Autodesk Inventor part; units mm, degrees
(part 2 of 2)
sketch "Sketch26" plane through (0, 0, 0) normal (0, -1, 0) x (1, 0, 0)
  circle A0 centre (0, 0) radius 23.8125 construction
  spline S0 degree 2 poles (-25.008, 3.6624) (-24.6681, 3.636) (-24.1674, 3.3369) (-24.0142, 3.1094) knots 0 0 0 1 2 2 2
  spline S1 degree 2 poles (-24.0142, 3.1094) (-23.8348, 2.8353) (-23.7106, 2.2348) (-23.7468, 1.7694) knots 0 0 0 1 2 2 2
  line L0 (-23.7468, 1.7694) -> (-23.8485, 0.4617)
  line L1 (-23.8485, 0.4617) -> (-28.4068, 0.8163)
  line L2 (-28.4068, 0.8163) -> (-28.3128, 2.0242)
  spline S2 degree 2 poles (-28.3128, 2.0242) (-28.2749, 2.5118) (-28.1741, 2.9945) (-28.035, 3.2067) knots 0 0 0 1 2 2 2
  spline S3 degree 2 poles (-28.035, 3.2067) (-27.8864, 3.4441) (-27.4441, 3.6364) (-27.156, 3.614) knots 0 0 0 1 2 2 2
  spline S4 degree 2 poles (-27.156, 3.614) (-26.8346, 3.589) (-26.3513, 3.2095) (-26.2305, 2.8991) knots 0 0 0 1 2 2 2
  line L3 (-26.2305, 2.8991) -> (-26.2084, 2.8973)
  spline S5 degree 2 poles (-26.2084, 2.8973) (-26.0659, 3.2951) (-25.4439, 3.6963) (-25.008, 3.6624) knots 0 0 0 1 2 2 2
  spline S6 degree 2 poles (-25.0313, 3.0287) (-25.2898, 3.0489) (-25.6338, 2.927) (-25.7692, 2.7145) knots 0 0 0 1 2 2 2
  spline S7 degree 2 poles (-25.7692, 2.7145) (-25.8543, 2.5762) (-25.9251, 2.2398) (-25.9495, 1.9259) knots 0 0 0 1 2 2 2
  line L4 (-25.9495, 1.9259) -> (-26.0029, 1.2388)
  line L5 (-26.0029, 1.2388) -> (-24.3185, 1.1078)
  line L6 (-24.3185, 1.1078) -> (-24.2803, 1.599)
  spline S8 degree 2 poles (-24.2803, 1.599) (-24.2493, 1.998) (-24.2875, 2.4618) (-24.3919, 2.6483) knots 0 0 0 1 2 2 2
  spline S9 degree 2 poles (-24.3919, 2.6483) (-24.5006, 2.8277) (-24.7912, 3.0101) (-25.0313, 3.0287) knots 0 0 0 1 2 2 2
  spline S10 degree 2 poles (-27.1202, 2.9757) (-27.2827, 2.9884) (-27.5351, 2.8965) (-27.6148, 2.7801) knots 0 0 0 1 2 2 2
  spline S11 degree 2 poles (-27.6148, 2.7801) (-27.7076, 2.6386) (-27.7724, 2.2832) (-27.7974, 1.9618) knots 0 0 0 1 2 2 2
  line L7 (-27.7974, 1.9618) -> (-27.8425, 1.3819)
  line L8 (-27.8425, 1.3819) -> (-26.509, 1.2782)
  line L9 (-26.509, 1.2782) -> (-26.4556, 1.9652)
  spline S12 degree 2 poles (-26.4556, 1.9652) (-26.4334, 2.2497) (-26.4715, 2.5239) (-26.5527, 2.6751) knots 0 0 0 1 2 2 2
  spline S13 degree 2 poles (-26.5527, 2.6751) (-26.6304, 2.8224) (-26.9059, 2.959) (-27.1202, 2.9757) knots 0 0 0 1 2 2 2
  spline S14 degree 2 poles (-24.5296, 7.2332) (-23.6849, 7.0382) (-22.9517, 6.0135) (-23.1084, 5.3348) knots 0 0 0 1 2 2 2
  spline S15 degree 2 poles (-23.1084, 5.3348) (-23.2692, 4.638) (-24.4028, 4.0593) (-25.2186, 4.2476) knots 0 0 0 1 2 2 2
  spline S16 degree 2 poles (-25.2186, 4.2476) (-26.0562, 4.4409) (-26.794, 5.4781) (-26.6391, 6.1496) knots 0 0 0 1 2 2 2
  spline S17 degree 2 poles (-26.6391, 6.1496) (-26.4825, 6.8283) (-25.3708, 7.4273) (-24.5296, 7.2332) knots 0 0 0 1 2 2 2
  spline S18 degree 2 poles (-24.6638, 6.6519) (-25.3136, 6.8019) (-26.0545, 6.4748) (-26.1553, 6.038) knots 0 0 0 1 2 2 2
  spline S19 degree 2 poles (-26.1553, 6.038) (-26.2561, 5.6011) (-25.7343, 4.9788) (-25.0845, 4.8288) knots 0 0 0 1 2 2 2
  spline S20 degree 2 poles (-25.0845, 4.8288) (-24.4527, 4.683) (-23.6929, 5.0096) (-23.5921, 5.4464) knots 0 0 0 1 2 2 2
  spline S21 degree 2 poles (-23.5921, 5.4464) (-23.4922, 5.8796) (-24.0212, 6.5036) (-24.6638, 6.6519) knots 0 0 0 1 2 2 2
  spline S22 degree 2 poles (-22.231, 8.3551) (-22.3891, 7.9119) (-23.073, 7.5933) (-23.6209, 7.7886) knots 0 0 0 1 2 2 2
  line L10 (-23.6209, 7.7886) -> (-25.4112, 8.4269)
  line L11 (-25.4112, 8.4269) -> (-25.5419, 8.0605)
  line L12 (-25.5419, 8.0605) -> (-25.992, 8.221)
  line L13 (-25.992, 8.221) -> (-25.8614, 8.5875)
  line L14 (-25.8614, 8.5875) -> (-26.7897, 8.9184)
  line L15 (-26.7897, 8.9184) -> (-26.5956, 9.4628)
  line L16 (-26.5956, 9.4628) -> (-25.6673, 9.1319)
  line L17 (-25.6673, 9.1319) -> (-25.3102, 10.1335)
  line L18 (-25.3102, 10.1335) -> (-24.86, 9.9729)
  line L19 (-24.86, 9.9729) -> (-25.2171, 8.9714)
  line L20 (-25.2171, 8.9714) -> (-23.6781, 8.4226)
  spline S23 degree 2 poles (-23.6781, 8.4226) (-23.4338, 8.3355) (-23.1589, 8.2572) (-23.0225, 8.2754) knots 0 0 0 1 2 2 2
  spline S24 degree 2 poles (-23.0225, 8.2754) (-22.9039, 8.2882) (-22.7243, 8.472) (-22.6571, 8.6604) knots 0 0 0 1 2 2 2
  spline S25 degree 2 poles (-22.6571, 8.6604) (-22.6098, 8.793) (-22.6018, 9.0694) (-22.6063, 9.134) knots 0 0 0 1 2 2 2
  line L21 (-22.6063, 9.134) -> (-22.5951, 9.1654)
  line L22 (-22.5951, 9.1654) -> (-22.1065, 8.9912)
  spline S26 degree 2 poles (-22.1065, 8.9912) (-22.1194, 8.8227) (-22.1825, 8.4912) (-22.231, 8.3551) knots 0 0 0 1 2 2 2
  spline S27 degree 2 poles (-21.4074, 10.2834) (-21.6039, 9.8559) (-22.3133, 9.5988) (-22.8419, 9.8417) knots 0 0 0 1 2 2 2
  line L23 (-22.8419, 9.8417) -> (-24.5689, 10.6355)
  line L24 (-24.5689, 10.6355) -> (-24.7313, 10.282)
  line L25 (-24.7313, 10.282) -> (-25.1656, 10.4816)
  line L26 (-25.1656, 10.4816) -> (-25.0032, 10.8351)
  line L27 (-25.0032, 10.8351) -> (-25.8986, 11.2466)
  line L28 (-25.8986, 11.2466) -> (-25.6573, 11.7718)
  line L29 (-25.6573, 11.7718) -> (-24.7618, 11.3602)
  line L30 (-24.7618, 11.3602) -> (-24.3177, 12.3264)
  line L31 (-24.3177, 12.3264) -> (-23.8834, 12.1268)
  line L32 (-23.8834, 12.1268) -> (-24.3275, 11.1606)
  line L33 (-24.3275, 11.1606) -> (-22.8429, 10.4783)
  spline S28 degree 2 poles (-22.8429, 10.4783) (-22.6072, 10.37) (-22.3403, 10.2677) (-22.2029, 10.2739) knots 0 0 0 1 2 2 2
  spline S29 degree 2 poles (-22.2029, 10.2739) (-22.0836, 10.2761) (-21.8885, 10.4433) (-21.8049, 10.6251) knots 0 0 0 1 2 2 2
  spline S30 degree 2 poles (-21.8049, 10.6251) (-21.7461, 10.7531) (-21.7137, 11.0277) (-21.7125, 11.0924) knots 0 0 0 1 2 2 2
  line L34 (-21.7125, 11.0924) -> (-21.6986, 11.1227)
  line L35 (-21.6986, 11.1227) -> (-21.2273, 10.906)
  spline S31 degree 2 poles (-21.2273, 10.906) (-21.255, 10.7393) (-21.3471, 10.4147) (-21.4074, 10.2834) knots 0 0 0 1 2 2 2
  spline S32 degree 2 poles (-21.0136, 14.5757) (-20.2729, 14.1252) (-19.8989, 12.922) (-20.2609, 12.3269) knots 0 0 0 1 2 2 2
  spline S33 degree 2 poles (-20.2609, 12.3269) (-20.6325, 11.7159) (-21.8906, 11.5228) (-22.606, 11.958) knots 0 0 0 1 2 2 2
  spline S34 degree 2 poles (-22.606, 11.958) (-23.3403, 12.4047) (-23.7148, 13.6212) (-23.3567, 14.21) knots 0 0 0 1 2 2 2
  spline S35 degree 2 poles (-23.3567, 14.21) (-22.9947, 14.8051) (-21.7511, 15.0244) (-21.0136, 14.5757) knots 0 0 0 1 2 2 2
  spline S36 degree 2 poles (-21.3236, 14.0661) (-21.8933, 14.4127) (-22.6995, 14.335) (-22.9325, 13.952) knots 0 0 0 1 2 2 2
  spline S37 degree 2 poles (-22.9325, 13.952) (-23.1655, 13.569) (-22.8657, 12.8142) (-22.296, 12.4676) knots 0 0 0 1 2 2 2
  spline S38 degree 2 poles (-22.296, 12.4676) (-21.742, 12.1306) (-20.9181, 12.2019) (-20.6851, 12.5849) knots 0 0 0 1 2 2 2
  spline S39 degree 2 poles (-20.6851, 12.5849) (-20.454, 12.9647) (-20.7601, 13.7234) (-21.3236, 14.0661) knots 0 0 0 1 2 2 2
  line L36 (-16.6582, 17.0976) -> (-18.1401, 18.4196)
  spline S40 degree 2 poles (-18.1401, 18.4196) (-18.317, 18.5774) (-18.643, 18.8186) (-18.7654, 18.8484) knots 0 0 0 1 2 2 2
  spline S41 degree 2 poles (-18.7654, 18.8484) (-18.8961, 18.8855) (-19.1351, 18.7958) (-19.2658, 18.6493) knots 0 0 0 1 2 2 2
  spline S42 degree 2 poles (-19.2658, 18.6493) (-19.3842, 18.5166) (-19.4924, 18.0669) (-19.4806, 17.7685) knots 0 0 0 1 2 2 2
  spline S43 degree 2 poles (-19.4806, 17.7685) (-19.4394, 17.7367) (-19.3267, 17.646) (-19.2548, 17.5819) knots 0 0 0 1 2 2 2
  line L37 (-19.2548, 17.5819) -> (-17.5683, 16.0774)
  line L38 (-17.5683, 16.0774) -> (-17.953, 15.6461)
  line L39 (-17.953, 15.6461) -> (-19.435, 16.9681)
  spline S44 degree 2 poles (-19.435, 16.9681) (-19.6119, 17.1259) (-19.9379, 17.3671) (-20.0603, 17.3969) knots 0 0 0 1 2 2 2
  spline S45 degree 2 poles (-20.0603, 17.3969) (-20.191, 17.434) (-20.43, 17.3443) (-20.5607, 17.1978) knots 0 0 0 1 2 2 2
  spline S46 degree 2 poles (-20.5607, 17.1978) (-20.684, 17.0595) (-20.7836, 16.5973) (-20.7764, 16.3327) knots 0 0 0 1 2 2 2
  line L40 (-20.7764, 16.3327) -> (-18.8632, 14.6259)
  line L41 (-18.8632, 14.6259) -> (-19.2479, 14.1946)
  line L42 (-19.2479, 14.1946) -> (-21.8081, 16.4785)
  line L43 (-21.8081, 16.4785) -> (-21.4233, 16.9098)
  line L44 (-21.4233, 16.9098) -> (-21.1413, 16.6582)
  spline S47 degree 2 poles (-21.1413, 16.6582) (-21.1595, 16.9773) (-21.0488, 17.4743) (-20.8712, 17.6734) knots 0 0 0 1 2 2 2
  spline S48 degree 2 poles (-20.8712, 17.6734) (-20.669, 17.9001) (-20.1484, 18.0663) (-19.832, 17.9478) knots 0 0 0 1 2 2 2
  spline S49 degree 2 poles (-19.832, 17.9478) (-19.8753, 18.339) (-19.7687, 18.9093) (-19.5763, 19.1249) knots 0 0 0 1 2 2 2
  spline S50 degree 2 poles (-19.5763, 19.1249) (-19.4283, 19.2908) (-19.0843, 19.4705) (-18.8794, 19.4664) knots 0 0 0 1 2 2 2
  spline S51 degree 2 poles (-18.8794, 19.4664) (-18.672, 19.4651) (-18.2226, 19.2677) (-17.9599, 19.0334) knots 0 0 0 1 2 2 2
  line L45 (-17.9599, 19.0334) -> (-16.2734, 17.5289)
  line L46 (-16.2734, 17.5289) -> (-16.6582, 17.0976)
  line L47 (-11.2556, 21.05) -> (-11.7702, 20.7269)
  line L48 (-11.7702, 20.7269) -> (-12.96, 22.6222)
  line L49 (-12.96, 22.6222) -> (-14.7424, 21.5032)
  line L50 (-14.7424, 21.5032) -> (-13.5525, 19.608)
  line L51 (-13.5525, 19.608) -> (-14.0671, 19.2849)
  line L52 (-14.0671, 19.2849) -> (-16.4981, 23.157)
  line L53 (-16.4981, 23.157) -> (-15.9835, 23.4801)
  line L54 (-15.9835, 23.4801) -> (-15.03, 21.9614)
  line L55 (-15.03, 21.9614) -> (-13.2477, 23.0803)
  line L56 (-13.2477, 23.0803) -> (-14.2011, 24.5991)
  line L57 (-14.2011, 24.5991) -> (-13.6865, 24.9222)
  line L58 (-13.6865, 24.9222) -> (-11.2556, 21.05)
  spline S52 degree 2 poles (-9.0603, 21.9388) (-9.8171, 21.6167) (-11.0102, 22.1116) (-11.3439, 22.8957) knots 0 0 0 1 2 2 2
  spline S53 degree 2 poles (-11.3439, 22.8957) (-11.6718, 23.6662) (-11.2526, 24.9237) (-10.6015, 25.2008) knots 0 0 0 1 2 2 2
  spline S54 degree 2 poles (-10.6015, 25.2008) (-10.3083, 25.3256) (-9.7823, 25.3481) (-9.5384, 25.2385) knots 0 0 0 1 2 2 2
  spline S55 degree 2 poles (-9.5384, 25.2385) (-9.291, 25.1303) (-8.8884, 24.6856) (-8.7273, 24.3072) knots 0 0 0 1 2 2 2
  line L59 (-8.7273, 24.3072) -> (-8.604, 24.0174)
  line L60 (-8.604, 24.0174) -> (-10.7893, 23.0875)
  spline S56 degree 2 poles (-10.7893, 23.0875) (-10.5557, 22.5386) (-9.7553, 22.1906) (-9.2644, 22.3996) knots 0 0 0 1 2 2 2
  spline S57 degree 2 poles (-9.2644, 22.3996) (-9.0906, 22.4735) (-8.7864, 22.6956) (-8.6762, 22.815) knots 0 0 0 1 2 2 2
  spline S58 degree 2 poles (-8.6762, 22.815) (-8.562, 22.9441) (-8.415, 23.1476) (-8.3735, 23.2297) knots 0 0 0 1 2 2 2
  line L61 (-8.3735, 23.2297) -> (-8.3428, 23.2427)
  line L62 (-8.3428, 23.2427) -> (-8.0962, 22.6632)
  spline S59 degree 2 poles (-8.0962, 22.6632) (-8.1722, 22.5865) (-8.4054, 22.3584) (-8.5014, 22.2813) knots 0 0 0 1 2 2 2
  spline S60 degree 2 poles (-8.5014, 22.2813) (-8.636, 22.1717) (-8.8694, 22.02) (-9.0603, 21.9388) knots 0 0 0 1 2 2 2
  spline S61 degree 2 poles (-9.2948, 24.2026) (-9.3931, 24.4145) (-9.6152, 24.6904) (-9.7454, 24.7598) knots 0 0 0 1 2 2 2
  spline S62 degree 2 poles (-9.7454, 24.7598) (-9.8882, 24.8399) (-10.2317, 24.8428) (-10.4464, 24.7514) knots 0 0 0 1 2 2 2
  spline S63 degree 2 poles (-10.4464, 24.7514) (-10.6578, 24.6614) (-10.9007, 24.4091) (-10.9712, 24.2341) knots 0 0 0 1 2 2 2
  spline S64 degree 2 poles (-10.9712, 24.2341) (-11.0369, 24.0572) (-11.0305, 23.7015) (-10.9619, 23.4931) knots 0 0 0 1 2 2 2
  line L63 (-10.9619, 23.4931) -> (-9.2948, 24.2026)
  line L64 (-4.8272, 23.368) -> (-5.5096, 23.1808)
  line L65 (-5.5096, 23.1808) -> (-6.6546, 24.2037)
  line L66 (-6.6546, 24.2037) -> (-7.1389, 22.7339)
  line L67 (-7.1389, 22.7339) -> (-7.7714, 22.5604)
  line L68 (-7.7714, 22.5604) -> (-7.0743, 24.515)
  line L69 (-7.0743, 24.515) -> (-8.6682, 25.872)
  line L70 (-8.6682, 25.872) -> (-7.9858, 26.0592)
  line L71 (-7.9858, 26.0592) -> (-6.8473, 25.046)
  line L72 (-6.8473, 25.046) -> (-6.3672, 26.5032)
  line L73 (-6.3672, 26.5032) -> (-5.7348, 26.6766)
  line L74 (-5.7348, 26.6766) -> (-6.4266, 24.7311)
  line L75 (-6.4266, 24.7311) -> (-4.8272, 23.368)
  line L76 (-3.7299, 26.1064) -> (-4.4546, 25.9926)
  line L77 (-4.4546, 25.9926) -> (-4.5903, 26.8563)
  line L78 (-4.5903, 26.8563) -> (-3.8656, 26.9702)
  line L79 (-3.8656, 26.9702) -> (-3.7299, 26.1064)
  line L80 (-3.3332, 23.5809) -> (-4.0579, 23.4671)
  line L81 (-4.0579, 23.4671) -> (-4.1936, 24.3309)
  line L82 (-4.1936, 24.3309) -> (-3.4689, 24.4447)
  line L83 (-3.4689, 24.4447) -> (-3.3332, 23.5809)
  spline S65 degree 2 poles (2.64, 26.0058) (2.5845, 24.777) (1.8181, 23.6582) (1.0742, 23.6918) knots 0 0 0 1 2 2 2
  spline S66 degree 2 poles (1.0742, 23.6918) (0.3191, 23.7259) (-0.3348, 24.9312) (-0.2805, 26.1341) knots 0 0 0 1 2 2 2
  spline S67 degree 2 poles (-0.2805, 26.1341) (-0.2246, 27.3703) (0.5414, 28.4817) (1.2891, 28.4479) knots 0 0 0 1 2 2 2
  spline S68 degree 2 poles (1.2891, 28.4479) (2.0404, 28.414) (2.6938, 27.1976) (2.64, 26.0058) knots 0 0 0 1 2 2 2
  spline S69 degree 2 poles (1.7924, 24.6496) (1.8915, 24.8714) (1.9969, 25.5639) (2.0182, 26.0339) knots 0 0 0 1 2 2 2
  spline S70 degree 2 poles (2.0182, 26.0339) (2.0394, 26.504) (1.9967, 27.1995) (1.9147, 27.4368) knots 0 0 0 1 2 2 2
  spline S71 degree 2 poles (1.9147, 27.4368) (1.8327, 27.6742) (1.5215, 27.9293) (1.2661, 27.9409) knots 0 0 0 1 2 2 2
  spline S72 degree 2 poles (1.2661, 27.9409) (1.0108, 27.9524) (0.6705, 27.7267) (0.5634, 27.4905) knots 0 0 0 1 2 2 2
  spline S73 degree 2 poles (0.5634, 27.4905) (0.4603, 27.2615) (0.3616, 26.5538) (0.3413, 26.106) knots 0 0 0 1 2 2 2
  spline S74 degree 2 poles (0.3413, 26.106) (0.3196, 25.6248) (0.3497, 24.9781) (0.4346, 24.7221) knots 0 0 0 1 2 2 2
  spline S75 degree 2 poles (0.4346, 24.7221) (0.5127, 24.4812) (0.8306, 24.2109) (1.0971, 24.1989) knots 0 0 0 1 2 2 2
  spline S76 degree 2 poles (1.0971, 24.1989) (1.3488, 24.1875) (1.689, 24.4132) (1.7924, 24.6496) knots 0 0 0 1 2 2 2
  line L84 (4.0826, 23.4627) -> (3.358, 23.5774)
  line L85 (3.358, 23.5774) -> (3.4948, 24.4411)
  line L86 (3.4948, 24.4411) -> (4.2193, 24.3263)
  line L87 (4.2193, 24.3263) -> (4.0826, 23.4627)
  spline S77 degree 2 poles (8.0519, 23.9877) (7.9643, 23.6698) (7.6111, 23.183) (7.3702, 23.0342) knots 0 0 0 1 2 2 2
  spline S78 degree 2 poles (7.3702, 23.0342) (7.1294, 22.8853) (6.5117, 22.8057) (6.1688, 22.9002) knots 0 0 0 1 2 2 2
  spline S79 degree 2 poles (6.1688, 22.9002) (5.8545, 22.9869) (5.2785, 23.2955) (5.084, 23.4682) knots 0 0 0 1 2 2 2
  line L88 (5.084, 23.4682) -> (5.2563, 24.0933)
  line L89 (5.2563, 24.0933) -> (5.2991, 24.0815)
  spline S80 degree 2 poles (5.2991, 24.0815) (5.3532, 24.0128) (5.5714, 23.8143) (5.7092, 23.7148) knots 0 0 0 1 2 2 2
  spline S81 degree 2 poles (5.7092, 23.7148) (5.8675, 23.6059) (6.1381, 23.4583) (6.3203, 23.4081) knots 0 0 0 1 2 2 2
  spline S82 degree 2 poles (6.3203, 23.4081) (6.4989, 23.3588) (6.8701, 23.3949) (7.0299, 23.5007) knots 0 0 0 1 2 2 2
  spline S83 degree 2 poles (7.0299, 23.5007) (7.1771, 23.6024) (7.3878, 23.9209) (7.4528, 24.1567) knots 0 0 0 1 2 2 2
  spline S84 degree 2 poles (7.4528, 24.1567) (7.5178, 24.3924) (7.4719, 24.7279) (7.378, 24.8614) knots 0 0 0 1 2 2 2
  spline S85 degree 2 poles (7.378, 24.8614) (7.2835, 25.0065) (6.9376, 25.2018) (6.7126, 25.2638) knots 0 0 0 1 2 2 2
  spline S86 degree 2 poles (6.7126, 25.2638) (6.4697, 25.3307) (5.9668, 25.3886) (5.8115, 25.3968) knots 0 0 0 1 2 2 2
  line L90 (5.8115, 25.3968) -> (6.4376, 27.6685)
  line L91 (6.4376, 27.6685) -> (8.8557, 27.0021)
  line L92 (8.8557, 27.0021) -> (8.713, 26.4842)
  line L93 (8.713, 26.4842) -> (6.8628, 26.9941)
  line L94 (6.8628, 26.9941) -> (6.5389, 25.819)
  spline S87 degree 2 poles (6.5389, 25.819) (6.65, 25.8037) (6.8601, 25.7573) (6.9459, 25.7337) knots 0 0 0 1 2 2 2
  spline S88 degree 2 poles (6.9459, 25.7337) (7.2852, 25.6402) (7.7226, 25.4005) (7.8916, 25.1772) knots 0 0 0 1 2 2 2
  spline S89 degree 2 poles (7.8916, 25.1772) (8.0642, 24.9528) (8.1622, 24.3878) (8.0519, 23.9877) knots 0 0 0 1 2 2 2
  line L95 (11.6107, 22.6262) -> (11.1118, 22.8446)
  line L96 (11.1118, 22.8446) -> (10.4817, 21.4056)
  line L97 (10.4817, 21.4056) -> (9.942, 21.6419)
  line L98 (9.942, 21.6419) -> (10.5722, 23.0809)
  line L99 (10.5722, 23.0809) -> (8.7225, 23.8909)
  line L100 (8.7225, 23.8909) -> (8.9811, 24.4814)
  line L101 (8.9811, 24.4814) -> (11.7997, 25.8196)
  line L102 (11.7997, 25.8196) -> (12.3156, 25.5937)
  line L103 (12.3156, 25.5937) -> (11.3095, 23.296)
  line L104 (11.3095, 23.296) -> (11.8084, 23.0776)
  line L105 (11.8084, 23.0776) -> (11.6107, 22.6262)
  line L106 (10.7698, 23.5323) -> (11.4862, 25.1682)
  line L107 (11.4862, 25.1682) -> (9.3614, 24.1491)
  line L108 (9.3614, 24.1491) -> (10.7698, 23.5323)
  spline S90 degree 2 poles (15.0299, 21.3864) (14.38, 20.3419) (13.1642, 19.7414) (12.5319, 20.1348) knots 0 0 0 1 2 2 2
  spline S91 degree 2 poles (12.5319, 20.1348) (11.8901, 20.5341) (11.9097, 21.9051) (12.5458, 22.9275) knots 0 0 0 1 2 2 2
  spline S92 degree 2 poles (12.5458, 22.9275) (13.1996, 23.9782) (14.4115, 24.5725) (15.047, 24.1772) knots 0 0 0 1 2 2 2
  spline S93 degree 2 poles (15.047, 24.1772) (15.6856, 23.7798) (15.6601, 22.3993) (15.0299, 21.3864) knots 0 0 0 1 2 2 2
  spline S94 degree 2 poles (13.627, 20.6185) (13.8219, 20.7634) (14.2528, 21.3157) (14.5014, 21.7152) knots 0 0 0 1 2 2 2
  spline S95 degree 2 poles (14.5014, 21.7152) (14.7499, 22.1147) (15.053, 22.7421) (15.0977, 22.9892) knots 0 0 0 1 2 2 2
  spline S96 degree 2 poles (15.0977, 22.9892) (15.1424, 23.2364) (14.9959, 23.6111) (14.7788, 23.7462) knots 0 0 0 1 2 2 2
  spline S97 degree 2 poles (14.7788, 23.7462) (14.5618, 23.8812) (14.1546, 23.851) (13.9456, 23.6974) knots 0 0 0 1 2 2 2
  spline S98 degree 2 poles (13.9456, 23.6974) (13.7436, 23.5481) (13.3112, 22.9793) (13.0743, 22.5987) knots 0 0 0 1 2 2 2
  spline S99 degree 2 poles (13.0743, 22.5987) (12.8199, 22.1897) (12.5297, 21.611) (12.4784, 21.3462) knots 0 0 0 1 2 2 2
  spline S100 degree 2 poles (12.4784, 21.3462) (12.4286, 21.0979) (12.5735, 20.7067) (12.8, 20.5657) knots 0 0 0 1 2 2 2
  spline S101 degree 2 poles (12.8, 20.5657) (13.0139, 20.4326) (13.4211, 20.4629) (13.627, 20.6185) knots 0 0 0 1 2 2 2
  line L109 (17.0472, 16.6496) -> (15.7637, 17.8698)
  line L110 (15.7637, 17.8698) -> (16.0853, 18.2081)
  line L111 (16.0853, 18.2081) -> (16.5069, 17.8073)
  line L112 (16.5069, 17.8073) -> (19.0137, 20.4443)
  line L113 (19.0137, 20.4443) -> (18.5921, 20.845)
  line L114 (18.5921, 20.845) -> (18.9138, 21.1834)
  line L115 (18.9138, 21.1834) -> (20.1973, 19.9632)
  line L116 (20.1973, 19.9632) -> (19.8757, 19.6248)
  line L117 (19.8757, 19.6248) -> (19.4541, 20.0256)
  line L118 (19.4541, 20.0256) -> (16.9473, 17.3887)
  line L119 (16.9473, 17.3887) -> (17.3689, 16.9879)
  line L120 (17.3689, 16.9879) -> (17.0472, 16.6496)
  spline S102 degree 2 poles (21.6238, 14.7343) (21.1338, 14.3444) (20.0292, 14.114) (19.5436, 14.2721) knots 0 0 0 1 2 2 2
  spline S103 degree 2 poles (19.5436, 14.2721) (19.1557, 14.4085) (18.5944, 14.8757) (18.2484, 15.3106) knots 0 0 0 1 2 2 2
  line L121 (18.2484, 15.3106) -> (17.5931, 16.1339)
  line L122 (17.5931, 16.1339) -> (21.1706, 18.9808)
  line L123 (21.1706, 18.9808) -> (21.8189, 18.1662)
  spline S104 degree 2 poles (21.8189, 18.1662) (22.2203, 17.6618) (22.5264, 16.9678) (22.5545, 16.6587) knots 0 0 0 1 2 2 2
  spline S105 degree 2 poles (22.5545, 16.6587) (22.6, 16.1315) (22.1456, 15.1495) (21.6238, 14.7343) knots 0 0 0 1 2 2 2
  spline S106 degree 2 poles (21.235, 15.2346) (21.6467, 15.5622) (22.0126, 16.2985) (21.9632, 16.6996) knots 0 0 0 1 2 2 2
  spline S107 degree 2 poles (21.9632, 16.6996) (21.924, 16.9809) (21.6818, 17.4936) (21.4257, 17.8154) knots 0 0 0 1 2 2 2
  line L124 (21.4257, 17.8154) -> (21.1373, 18.1778)
  line L125 (21.1373, 18.1778) -> (18.3832, 15.986)
  line L126 (18.3832, 15.986) -> (18.6716, 15.6237)
  spline S108 degree 2 poles (18.6716, 15.6237) (18.923, 15.3077) (19.4052, 14.9101) (19.696, 14.8243) knots 0 0 0 1 2 2 2
  spline S109 degree 2 poles (19.696, 14.8243) (20.0626, 14.7088) (20.8176, 14.9024) (21.235, 15.2346) knots 0 0 0 1 2 2 2
  line L127 (20.6576, 11.8505) -> (20.2828, 12.4811)
  line L128 (20.2828, 12.4811) -> (21.0345, 12.9278)
  line L129 (21.0345, 12.9278) -> (21.4092, 12.2972)
  line L130 (21.4092, 12.2972) -> (20.6576, 11.8505)
  line L131 (22.8552, 13.1566) -> (22.4804, 13.7872)
  line L132 (22.4804, 13.7872) -> (23.2321, 14.2339)
  line L133 (23.2321, 14.2339) -> (23.6069, 13.6033)
  line L134 (23.6069, 13.6033) -> (22.8552, 13.1566)
  line L135 (22.8842, 6.694) -> (22.1503, 8.8002)
  line L136 (22.1503, 8.8002) -> (22.5912, 8.9538)
  line L137 (22.5912, 8.9538) -> (22.8642, 8.1701)
  line L138 (22.8642, 8.1701) -> (25.7577, 9.1782)
  line L139 (25.7577, 9.1782) -> (25.4846, 9.9619)
  line L140 (25.4846, 9.9619) -> (25.88, 10.0997)
  spline S110 degree 2 poles (25.88, 10.0997) (26.0348, 9.6553) (26.433, 9.3232) (26.7926, 9.4171) knots 0 0 0 1 2 2 2
  line L141 (26.7926, 9.4171) -> (26.9487, 8.9693)
  line L142 (26.9487, 8.9693) -> (23.058, 7.6138)
  line L143 (23.058, 7.6138) -> (23.325, 6.8476)
  line L144 (23.325, 6.8476) -> (22.8842, 6.694)
  line L145 (23.3013, 4.9209) -> (23.1388, 5.6363)
  line L146 (23.1388, 5.6363) -> (23.9915, 5.83)
  line L147 (23.9915, 5.83) -> (24.154, 5.1146)
  line L148 (24.154, 5.1146) -> (23.3013, 4.9209)
  spline S111 degree 2 poles (25.2626, 1.4303) (24.9349, 1.3936) (24.3517, 1.5408) (24.1241, 1.7092) knots 0 0 0 1 2 2 2
  spline S112 degree 2 poles (24.1241, 1.7092) (23.8965, 1.8776) (23.5932, 2.4215) (23.5537, 2.775) knots 0 0 0 1 2 2 2
  spline S113 degree 2 poles (23.5537, 2.775) (23.5174, 3.099) (23.5901, 3.7484) (23.6783, 3.9931) knots 0 0 0 1 2 2 2
  line L149 (23.6783, 3.9931) -> (24.3226, 4.0653)
  line L150 (24.3226, 4.0653) -> (24.3276, 4.0211)
  spline S114 degree 2 poles (24.3276, 4.0211) (24.2838, 3.9454) (24.1806, 3.6691) (24.1394, 3.5042) knots 0 0 0 1 2 2 2
  spline S115 degree 2 poles (24.1394, 3.5042) (24.097, 3.3167) (24.0604, 3.0107) (24.0814, 2.8229) knots 0 0 0 1 2 2 2
  spline S116 degree 2 poles (24.0814, 2.8229) (24.102, 2.6388) (24.2733, 2.3075) (24.431, 2.1984) knots 0 0 0 1 2 2 2
  spline S117 degree 2 poles (24.431, 2.1984) (24.58, 2.0995) (24.954, 2.0221) (25.197, 2.0493) knots 0 0 0 1 2 2 2
  spline S118 degree 2 poles (25.197, 2.0493) (25.44, 2.0765) (25.7345, 2.2437) (25.8236, 2.3804) knots 0 0 0 1 2 2 2
  spline S119 degree 2 poles (25.8236, 2.3804) (25.9233, 2.5221) (25.9761, 2.9157) (25.9502, 3.1477) knots 0 0 0 1 2 2 2
  spline S120 degree 2 poles (25.9502, 3.1477) (25.9221, 3.3981) (25.7892, 3.8865) (25.7391, 4.0337) knots 0 0 0 1 2 2 2
  line L151 (25.7391, 4.0337) -> (28.0809, 4.2959)
  line L152 (28.0809, 4.2959) -> (28.36, 1.8032)
  line L153 (28.36, 1.8032) -> (27.8261, 1.7434)
  line L154 (27.8261, 1.7434) -> (27.6125, 3.6507)
  line L155 (27.6125, 3.6507) -> (26.4011, 3.5151)
  spline S121 degree 2 poles (26.4011, 3.5151) (26.4282, 3.4063) (26.4632, 3.1939) (26.4731, 3.1056) knots 0 0 0 1 2 2 2
  spline S122 degree 2 poles (26.4731, 3.1056) (26.5123, 2.7558) (26.4521, 2.2607) (26.3075, 2.0208) knots 0 0 0 1 2 2 2
  spline S123 degree 2 poles (26.3075, 2.0208) (26.1632, 1.7772) (25.675, 1.4765) (25.2626, 1.4303) knots 0 0 0 1 2 2 2
  line L156 (28.589, -0.139) -> (26.8125, 0.0181)
  line L157 (26.8125, 0.0181) -> (26.8179, 0.4219)
  line L158 (26.8179, 0.4219) -> (28.5979, 0.5316)
  line L159 (28.5979, 0.5316) -> (28.589, -0.139)
  line L160 (28.5735, -1.2948) -> (26.7971, -1.1377)
  line L161 (26.7971, -1.1377) -> (26.8025, -0.7339)
  line L162 (26.8025, -0.7339) -> (28.5825, -0.6243)
  line L163 (28.5825, -0.6243) -> (28.5735, -1.2948)
  spline S124 degree 2 poles (26.6984, -8.103) (26.3413, -8.2821) (25.4088, -8.3497) (24.8548, -8.213) knots 0 0 0 1 2 2 2
  spline S125 degree 2 poles (24.8548, -8.213) (24.3152, -8.0799) (23.5086, -7.5909) (23.2775, -7.2592) knots 0 0 0 1 2 2 2
  spline S126 degree 2 poles (23.2775, -7.2592) (23.0356, -6.9095) (22.919, -6.1137) (23.0263, -5.6784) knots 0 0 0 1 2 2 2
  spline S127 degree 2 poles (23.0263, -5.6784) (23.1373, -5.2287) (23.6205, -4.5847) (23.9838, -4.3958) knots 0 0 0 1 2 2 2
  spline S128 degree 2 poles (23.9838, -4.3958) (24.3418, -4.2132) (25.2762, -4.1536) (25.823, -4.2885) knots 0 0 0 1 2 2 2
  spline S129 degree 2 poles (25.823, -4.2885) (26.3805, -4.4261) (27.1611, -4.9125) (27.4039, -5.2433) knots 0 0 0 1 2 2 2
  spline S130 degree 2 poles (27.4039, -5.2433) (27.635, -5.575) (27.7624, -6.3735) (27.6523, -6.8196) knots 0 0 0 1 2 2 2
  spline S131 degree 2 poles (27.6523, -6.8196) (27.5405, -7.2728) (27.0447, -7.9213) (26.6984, -8.103) knots 0 0 0 1 2 2 2
  spline S132 degree 2 poles (25.0066, -7.5979) (25.4454, -7.7062) (26.1723, -7.6832) (26.4379, -7.5656) knots 0 0 0 1 2 2 2
  spline S133 degree 2 poles (26.4379, -7.5656) (26.7116, -7.4461) (27.0643, -7.0065) (27.1406, -6.6972) knots 0 0 0 1 2 2 2
  spline S134 degree 2 poles (27.1406, -6.6972) (27.2196, -6.377) (27.1155, -5.84) (26.9233, -5.5979) knots 0 0 0 1 2 2 2
  spline S135 degree 2 poles (26.9233, -5.5979) (26.7402, -5.3658) (26.1029, -5.0101) (25.6712, -4.9036) knots 0 0 0 1 2 2 2
  spline S136 degree 2 poles (25.6712, -4.9036) (24.7971, -4.688) (23.688, -5.1929) (23.5363, -5.808) knots 0 0 0 1 2 2 2
  spline S137 degree 2 poles (23.5363, -5.808) (23.3845, -6.4231) (24.1325, -7.3823) (25.0066, -7.5979) knots 0 0 0 1 2 2 2
  spline S138 degree 2 poles (22.9836, -12.5076) (22.413, -12.2498) (21.7036, -11.3723) (21.6224, -10.8681) knots 0 0 0 1 2 2 2
  spline S139 degree 2 poles (21.6224, -10.8681) (21.5666, -10.4607) (21.7259, -9.748) (21.9547, -9.2416) knots 0 0 0 1 2 2 2
  line L164 (21.9547, -9.2416) -> (22.3879, -8.2827)
  line L165 (22.3879, -8.2827) -> (26.5545, -10.165)
  line L166 (26.5545, -10.165) -> (26.1258, -11.1138)
  spline S140 degree 2 poles (26.1258, -11.1138) (25.8604, -11.7013) (25.3828, -12.2905) (25.1207, -12.4567) knots 0 0 0 1 2 2 2
  spline S141 degree 2 poles (25.1207, -12.4567) (24.6725, -12.738) (23.5914, -12.7821) (22.9836, -12.5076) knots 0 0 0 1 2 2 2
  spline S142 degree 2 poles (23.2512, -11.9333) (23.7307, -12.1499) (24.5527, -12.1391) (24.887, -11.912) knots 0 0 0 1 2 2 2
  spline S143 degree 2 poles (24.887, -11.912) (25.1194, -11.7487) (25.4648, -11.299) (25.6342, -10.9242) knots 0 0 0 1 2 2 2
  line L167 (25.6342, -10.9242) -> (25.8248, -10.5021)
  line L168 (25.8248, -10.5021) -> (22.6172, -9.053)
  line L169 (22.6172, -9.053) -> (22.4265, -9.4751)
  spline S144 degree 2 poles (22.4265, -9.4751) (22.2603, -9.8431) (22.1268, -10.4536) (22.1833, -10.7515) knots 0 0 0 1 2 2 2
  spline S145 degree 2 poles (22.1833, -10.7515) (22.2479, -11.1304) (22.765, -11.7136) (23.2512, -11.9333) knots 0 0 0 1 2 2 2
  line L170 (19.9769, -12.9651) -> (20.3667, -12.3437)
  line L171 (20.3667, -12.3437) -> (21.1074, -12.8083)
  line L172 (21.1074, -12.8083) -> (20.7176, -13.4298)
  line L173 (20.7176, -13.4298) -> (19.9769, -12.9651)
  line L174 (22.1425, -14.3237) -> (22.5323, -13.7022)
  line L175 (22.5323, -13.7022) -> (23.273, -14.1669)
  line L176 (23.273, -14.1669) -> (22.8832, -14.7883)
  line L177 (22.8832, -14.7883) -> (22.1425, -14.3237)
  line L178 (16.248, -17.4672) -> (18.193, -15.426)
  line L179 (18.193, -15.426) -> (18.6624, -15.8732)
  spline S146 degree 2 poles (18.6624, -15.8732) (18.6594, -16.29) (18.6698, -17.0471) (18.6974, -17.4317) knots 0 0 0 1 2 2 2
  spline S147 degree 2 poles (18.6974, -17.4317) (18.7528, -18.206) (18.9885, -18.9577) (19.254, -19.2107) knots 0 0 0 1 2 2 2
  spline S148 degree 2 poles (19.254, -19.2107) (19.3935, -19.3436) (19.6845, -19.4571) (19.8257, -19.4432) knots 0 0 0 1 2 2 2
  spline S149 degree 2 poles (19.8257, -19.4432) (19.9669, -19.4293) (20.2282, -19.2894) (20.3457, -19.166) knots 0 0 0 1 2 2 2
  spline S150 degree 2 poles (20.3457, -19.166) (20.4582, -19.048) (20.6292, -18.7503) (20.6884, -18.5969) knots 0 0 0 1 2 2 2
  spline S151 degree 2 poles (20.6884, -18.5969) (20.7403, -18.4672) (20.7991, -18.1907) (20.8127, -18.1012) knots 0 0 0 1 2 2 2
  line L180 (20.8127, -18.1012) -> (20.8357, -18.0771)
  line L181 (20.8357, -18.0771) -> (21.3078, -18.5269)
  spline S152 degree 2 poles (21.3078, -18.5269) (21.2445, -18.7276) (20.9082, -19.3437) (20.6986, -19.5637) knots 0 0 0 1 2 2 2
  spline S153 degree 2 poles (20.6986, -19.5637) (20.2565, -20.0277) (19.2672, -20.0831) (18.8488, -19.6843) knots 0 0 0 1 2 2 2
  spline S154 degree 2 poles (18.8488, -19.6843) (18.653, -19.4978) (18.4126, -19.0948) (18.3498, -18.8814) knots 0 0 0 1 2 2 2
  spline S155 degree 2 poles (18.3498, -18.8814) (18.2816, -18.6629) (18.2197, -18.1586) (18.2056, -17.8995) knots 0 0 0 1 2 2 2
  spline S156 degree 2 poles (18.2056, -17.8995) (18.1769, -17.4731) (18.1769, -16.4956) (18.1804, -16.2072) knots 0 0 0 1 2 2 2
  line L182 (18.1804, -16.2072) -> (16.6316, -17.8327)
  line L183 (16.6316, -17.8327) -> (16.248, -17.4672)
  line L184 (15.0197, -18.4818) -> (15.5818, -18.0105)
  line L185 (15.5818, -18.0105) -> (16.1436, -18.6806)
  line L186 (16.1436, -18.6806) -> (15.5814, -19.1519)
  line L187 (15.5814, -19.1519) -> (15.0197, -18.4818)
  spline S157 degree 2 poles (12.8101, -21.8208) (12.6278, -21.546) (12.4924, -20.96) (12.5382, -20.6806) knots 0 0 0 1 2 2 2
  spline S158 degree 2 poles (12.5382, -20.6806) (12.5841, -20.4012) (12.9295, -19.883) (13.2258, -19.6864) knots 0 0 0 1 2 2 2
  spline S159 degree 2 poles (13.2258, -19.6864) (13.4975, -19.5061) (14.1084, -19.2742) (14.3664, -19.2409) knots 0 0 0 1 2 2 2
  line L188 (14.3664, -19.2409) -> (14.7249, -19.7811)
  line L189 (14.7249, -19.7811) -> (14.6878, -19.8057)
  spline S160 degree 2 poles (14.6878, -19.8057) (14.6005, -19.8014) (14.3076, -19.8357) (14.142, -19.8744) knots 0 0 0 1 2 2 2
  spline S161 degree 2 poles (14.142, -19.8744) (13.9559, -19.9223) (13.6669, -20.0295) (13.5095, -20.134) knots 0 0 0 1 2 2 2
  spline S162 degree 2 poles (13.5095, -20.134) (13.3551, -20.2364) (13.1387, -20.5401) (13.1136, -20.7301) knots 0 0 0 1 2 2 2
  spline S163 degree 2 poles (13.1136, -20.7301) (13.0937, -20.9079) (13.1956, -21.276) (13.3308, -21.4797) knots 0 0 0 1 2 2 2
  spline S164 degree 2 poles (13.3308, -21.4797) (13.466, -21.6835) (13.7492, -21.8691) (13.9115, -21.8859) knots 0 0 0 1 2 2 2
  spline S165 degree 2 poles (13.9115, -21.8859) (14.0831, -21.9099) (14.4574, -21.7772) (14.6519, -21.6481) knots 0 0 0 1 2 2 2
  spline S166 degree 2 poles (14.6519, -21.6481) (14.8618, -21.5088) (15.2356, -21.1675) (15.3438, -21.0557) knots 0 0 0 1 2 2 2
  line L190 (15.3438, -21.0557) -> (16.6465, -23.0192)
  line L191 (16.6465, -23.0192) -> (14.5564, -24.4059)
  line L192 (14.5564, -24.4059) -> (14.2594, -23.9583)
  line L193 (14.2594, -23.9583) -> (15.8586, -22.8972)
  line L194 (15.8586, -22.8972) -> (15.1847, -21.8815)
  spline S167 degree 2 poles (15.1847, -21.8815) (15.1003, -21.9553) (14.9274, -22.0834) (14.8533, -22.1325) knots 0 0 0 1 2 2 2
  spline S168 degree 2 poles (14.8533, -22.1325) (14.56, -22.3271) (14.092, -22.4998) (13.8126, -22.4807) knots 0 0 0 1 2 2 2
  spline S169 degree 2 poles (13.8126, -22.4807) (13.53, -22.4636) (13.0395, -22.1666) (12.8101, -21.8208) knots 0 0 0 1 2 2 2
  line L195 (11.8979, -26.0108) -> (11.2263, -24.3587)
  line L196 (11.2263, -24.3587) -> (11.588, -24.1791)
  line L197 (11.588, -24.1791) -> (12.4985, -25.7126)
  line L198 (12.4985, -25.7126) -> (11.8979, -26.0108)
  line L199 (12.9332, -25.4967) -> (12.2616, -23.8445)
  line L200 (12.2616, -23.8445) -> (12.6233, -23.6649)
  line L201 (12.6233, -23.6649) -> (13.5338, -25.1984)
  line L202 (13.5338, -25.1984) -> (12.9332, -25.4967)
  line L203 (3.9698, -23.5379) -> (4.5605, -23.3954)
  line L204 (4.5605, -23.3954) -> (5.0852, -25.5708)
  line L205 (5.0852, -25.5708) -> (7.131, -25.0774)
  line L206 (7.131, -25.0774) -> (6.6063, -22.9019)
  line L207 (6.6063, -22.9019) -> (7.197, -22.7595)
  line L208 (7.197, -22.7595) -> (8.269, -27.204)
  line L209 (8.269, -27.204) -> (7.6783, -27.3465)
  line L210 (7.6783, -27.3465) -> (7.2579, -25.6032)
  line L211 (7.2579, -25.6032) -> (5.2121, -26.0967)
  line L212 (5.2121, -26.0967) -> (5.6325, -27.8399)
  line L213 (5.6325, -27.8399) -> (5.0419, -27.9824)
  line L214 (5.0419, -27.9824) -> (3.9698, -23.5379)
  spline S170 degree 2 poles (2.054, -23.6603) (2.522, -23.6116) (3.1045, -24.0912) (3.1647, -24.6697) knots 0 0 0 1 2 2 2
  line L215 (3.1647, -24.6697) -> (3.3612, -26.5602)
  line L216 (3.3612, -26.5602) -> (3.7482, -26.52)
  line L217 (3.7482, -26.52) -> (3.7976, -26.9954)
  line L218 (3.7976, -26.9954) -> (3.4107, -27.0356)
  line L219 (3.4107, -27.0356) -> (3.5126, -28.0158)
  line L220 (3.5126, -28.0158) -> (2.9377, -28.0756)
  line L221 (2.9377, -28.0756) -> (2.8358, -27.0954)
  line L222 (2.8358, -27.0954) -> (1.7781, -27.2053)
  line L223 (1.7781, -27.2053) -> (1.7287, -26.7299)
  line L224 (1.7287, -26.7299) -> (2.7863, -26.62)
  line L225 (2.7863, -26.62) -> (2.6174, -24.9948)
  spline S171 degree 2 poles (2.6174, -24.9948) (2.5906, -24.7369) (2.5426, -24.455) (2.4673, -24.3399) knots 0 0 0 1 2 2 2
  spline S172 degree 2 poles (2.4673, -24.3399) (2.4046, -24.2384) (2.1614, -24.1557) (1.9624, -24.1764) knots 0 0 0 1 2 2 2
  spline S173 degree 2 poles (1.9624, -24.1764) (1.8223, -24.1909) (1.5695, -24.3029) (1.5132, -24.3348) knots 0 0 0 1 2 2 2
  line L226 (1.5132, -24.3348) -> (1.48, -24.3383)
  line L227 (1.48, -24.3383) -> (1.4264, -23.8224)
  spline S174 degree 2 poles (1.4264, -23.8224) (1.584, -23.7613) (1.9103, -23.6752) (2.054, -23.6603) knots 0 0 0 1 2 2 2
  line L228 (-0.0293, -26.3715) -> (0.7042, -26.3621)
  line L229 (0.7042, -26.3621) -> (0.7154, -27.2364)
  line L230 (0.7154, -27.2364) -> (-0.0182, -27.2458)
  line L231 (-0.0182, -27.2458) -> (-0.0293, -26.3715)
  line L232 (-0.0621, -23.8152) -> (0.6715, -23.8059)
  line L233 (0.6715, -23.8059) -> (0.6827, -24.6802)
  line L234 (0.6827, -24.6802) -> (-0.0509, -24.6896)
  line L235 (-0.0509, -24.6896) -> (-0.0621, -23.8152)
  spline S175 degree 2 poles (-5.0832, -27.4853) (-4.9194, -27.5165) (-4.5803, -27.4981) (-4.412, -27.466) knots 0 0 0 1 2 2 2
  spline S176 degree 2 poles (-4.412, -27.466) (-4.2546, -27.4319) (-4.0149, -27.3418) (-3.9201, -27.2995) knots 0 0 0 1 2 2 2
  line L236 (-3.9201, -27.2995) -> (-3.8837, -27.3064)
  line L237 (-3.8837, -27.3064) -> (-4.005, -27.9433)
  spline S177 degree 2 poles (-4.005, -27.9433) (-4.2216, -28.0114) (-4.9275, -28.0543) (-5.2296, -27.9968) knots 0 0 0 1 2 2 2
  spline S178 degree 2 poles (-5.2296, -27.9968) (-5.5354, -27.9385) (-5.9668, -27.7282) (-6.1274, -27.5618) knots 0 0 0 1 2 2 2
  spline S179 degree 2 poles (-6.1274, -27.5618) (-6.2969, -27.3824) (-6.4224, -26.9323) (-6.3698, -26.6557) knots 0 0 0 1 2 2 2
  spline S180 degree 2 poles (-6.3698, -26.6557) (-6.2991, -26.2845) (-5.7046, -25.8168) (-5.3486, -25.8092) knots 0 0 0 1 2 2 2
  line L238 (-5.3486, -25.8092) -> (-5.3403, -25.7655)
  spline S181 degree 2 poles (-5.3403, -25.7655) (-5.4767, -25.7094) (-5.7757, -25.5167) (-5.889, -25.3593) knots 0 0 0 1 2 2 2
  spline S182 degree 2 poles (-5.889, -25.3593) (-6.0031, -25.2056) (-6.1002, -24.7647) (-6.044, -24.4699) knots 0 0 0 1 2 2 2
  spline S183 degree 2 poles (-6.044, -24.4699) (-5.9865, -24.1678) (-5.6813, -23.6941) (-5.4546, -23.5336) knots 0 0 0 1 2 2 2
  spline S184 degree 2 poles (-5.4546, -23.5336) (-5.2193, -23.3672) (-4.6222, -23.2622) (-4.2692, -23.3294) knots 0 0 0 1 2 2 2
  spline S185 degree 2 poles (-4.2692, -23.3294) (-3.9307, -23.3938) (-3.2995, -23.6838) (-3.0953, -23.8396) knots 0 0 0 1 2 2 2
  line L239 (-3.0953, -23.8396) -> (-3.2166, -24.4765)
  line L240 (-3.2166, -24.4765) -> (-3.2603, -24.4682)
  spline S186 degree 2 poles (-3.2603, -24.4682) (-3.4232, -24.2938) (-4.0152, -23.9171) (-4.3319, -23.8568) knots 0 0 0 1 2 2 2
  spline S187 degree 2 poles (-4.3319, -23.8568) (-4.5175, -23.8214) (-4.9109, -23.8672) (-5.0603, -23.9783) knots 0 0 0 1 2 2 2
  spline S188 degree 2 poles (-5.0603, -23.9783) (-5.2061, -24.0901) (-5.3944, -24.3861) (-5.4409, -24.63) knots 0 0 0 1 2 2 2
  spline S189 degree 2 poles (-5.4409, -24.63) (-5.4873, -24.8738) (-5.4057, -25.2175) (-5.2956, -25.3328) knots 0 0 0 1 2 2 2
  spline S190 degree 2 poles (-5.2956, -25.3328) (-5.1856, -25.448) (-4.853, -25.583) (-4.6491, -25.6218) knots 0 0 0 1 2 2 2
  line L241 (-4.6491, -25.6218) -> (-4.3944, -25.6703)
  line L242 (-4.3944, -25.6703) -> (-4.4893, -26.169)
  line L243 (-4.4893, -26.169) -> (-4.6895, -26.1308)
  spline S191 degree 2 poles (-4.6895, -26.1308) (-5.0935, -26.0539) (-5.6765, -26.3427) (-5.7465, -26.7103) knots 0 0 0 1 2 2 2
  spline S192 degree 2 poles (-5.7465, -26.7103) (-5.7791, -26.8813) (-5.6945, -27.1501) (-5.6028, -27.243) knots 0 0 0 1 2 2 2
  spline S193 degree 2 poles (-5.6028, -27.243) (-5.5045, -27.341) (-5.2397, -27.4555) (-5.0832, -27.4853) knots 0 0 0 1 2 2 2
  line L244 (-7.3853, -22.6412) -> (-6.6845, -22.858)
  line L245 (-6.6845, -22.858) -> (-6.9429, -23.6934)
  line L246 (-6.9429, -23.6934) -> (-7.6437, -23.4765)
  line L247 (-7.6437, -23.4765) -> (-7.3853, -22.6412)
  spline S194 degree 2 poles (-11.7906, -23.3293) (-11.2981, -22.2021) (-10.1815, -21.4326) (-9.499, -21.7307) knots 0 0 0 1 2 2 2
  spline S195 degree 2 poles (-9.499, -21.7307) (-8.8064, -22.0334) (-8.6282, -23.3929) (-9.1104, -24.4963) knots 0 0 0 1 2 2 2
  spline S196 degree 2 poles (-9.1104, -24.4963) (-9.6058, -25.6303) (-10.7195, -26.3931) (-11.4053, -26.0934) knots 0 0 0 1 2 2 2
  spline S197 degree 2 poles (-11.4053, -26.0934) (-12.0945, -25.7923) (-12.2682, -24.4225) (-11.7906, -23.3293) knots 0 0 0 1 2 2 2
  spline S198 degree 2 poles (-10.513, -22.3672) (-10.685, -22.5387) (-11.0318, -23.1473) (-11.2202, -23.5785) knots 0 0 0 1 2 2 2
  spline S199 degree 2 poles (-11.2202, -23.5785) (-11.4086, -24.0097) (-11.6181, -24.6742) (-11.6267, -24.9252) knots 0 0 0 1 2 2 2
  spline S200 degree 2 poles (-11.6267, -24.9252) (-11.6352, -25.1762) (-11.4363, -25.5259) (-11.202, -25.6283) knots 0 0 0 1 2 2 2
  spline S201 degree 2 poles (-11.202, -25.6283) (-10.9678, -25.7306) (-10.5692, -25.642) (-10.3845, -25.4599) knots 0 0 0 1 2 2 2
  spline S202 degree 2 poles (-10.3845, -25.4599) (-10.2062, -25.2831) (-9.8602, -24.6579) (-9.6807, -24.2471) knots 0 0 0 1 2 2 2
  spline S203 degree 2 poles (-9.6807, -24.2471) (-9.4879, -23.8058) (-9.2841, -23.1913) (-9.2715, -22.9218) knots 0 0 0 1 2 2 2
  spline S204 degree 2 poles (-9.2715, -22.9218) (-9.258, -22.669) (-9.4578, -22.3027) (-9.7023, -22.1959) knots 0 0 0 1 2 2 2
  spline S205 degree 2 poles (-9.7023, -22.1959) (-9.9331, -22.095) (-10.3317, -22.1836) (-10.513, -22.3672) knots 0 0 0 1 2 2 2
  line L248 (-15.4042, -24.1005) -> (-14.3801, -22.6404)
  line L249 (-14.3801, -22.6404) -> (-14.0331, -22.847)
  line L250 (-14.0331, -22.847) -> (-14.8279, -24.4435)
  line L251 (-14.8279, -24.4435) -> (-15.4042, -24.1005)
  line L252 (-14.4108, -24.6917) -> (-13.3867, -23.2316)
  line L253 (-13.3867, -23.2316) -> (-13.0397, -23.4381)
  line L254 (-13.0397, -23.4381) -> (-13.8345, -25.0346)
  line L255 (-13.8345, -25.0346) -> (-14.4108, -24.6917)
  dimension "d145" = 47.625
  constraints: 1 centre point, 1 coincident, 1 other
  measures "d145" diameter of A0
extrude "Extrusion19" cut sketch "Sketch26" against normal blind 1.27
sketch "Sketch27" plane through (0, 72.39, 0) normal (0, 1, 0) x (1, 0, 0)
  line L0 (-3.9595, 6.858) -> (3.9595, 6.858)
  line L1 (3.9595, 6.858) -> (7.9189, 0)
  line L2 (7.9189, 0) -> (3.9595, -6.858)
  line L3 (3.9595, -6.858) -> (-3.9595, -6.858)
  line L4 (-3.9595, -6.858) -> (-7.9189, 0)
  line L5 (-7.9189, 0) -> (-3.9595, 6.858)
  point P0 (0, 0)
  point P1 (0, 0)
  dimension "d153" = 13.716
  constraints: 12 end point, 1 coincident, 1 horizontal, 13 other
  measures "d153" distance between parallel lines of L0 L3
extrude "Extrusion20" cut sketch "Sketch27" against normal through all
equation "\"d103\" = hexDiameter"
equation "\"d110\" = centerLineForSpool"
equation "\"d111\" = centerLineForSpool"
equation "\"d112\" = holeForString"
equation "\"d121\" = centerLineForSpool"
equation "\"d122\" = holeForString"
equation "\"d125\" = knotHoleDiameter"
equation "\"d127\" = holeForString"
equation "\"d128\" = centerLineForSpool"
equation "\"d129\" = knotHoleDiameter"
equation "\"d130\" = knotHoleDepth"
equation "\"d85\" = spoolExteriorRadius"
equation "\"d86\" = spoolOverallHeight"
equation "\"d88\" = d85"
equation "\"d89\" = 0.5 * spoolOverallHeight"
equation "\"centerLineForSpool\" = 0.25 * spoolOverallHeight"
equation "\"holeForString\" = stringDiameter + clearanceForString"
equation "\"stringDiameter\" = 3.048"
equation "\"clearanceForString\" = 2.032"
equation "\"hexShaftDiameter\" = 12.7"
equation "\"clearanceForHexShaft\" = 1.016"
equation "\"hexDiameter\" = hexShaftDiameter + clearanceForHexShaft"
equation "\"spoolInteriorDiameter\" = 38.1"
equation "\"spoolInteriroRadius\" = 0.5 * spoolInteriorDiameter"
equation "\"spoolExteriorDiameter\" = 63.5"
equation "\"spoolExteriorRadius\" = 0.5 * spoolExteriorDiameter"
equation "\"hexHoleChamfer\" = 1.5875"
equation "\"stringHoleCenterFromHexShaft\" = 0.5 * hexDiameter + 0.5 * holeForString"
equation "\"textCircleDiameter\" = 0.75 * spoolExteriorDiameter"
equation "\"textHeight\" = 4.572"
equation "\"textDepth\" = 1.27"
equation "\"spoolOverallHeight\" = 69.85"
equation "\"d114\" = -spoolInteriroRadius"
equation "\"knotHoleDiameter\" = 9.525"
equation "\"d126\" = spoolInteriroRadius"
equation "\"metalWasherID\" = 26.67"
equation "\"metalWasherThickness\" = 2.54"
equation "\"spacerOD\" = 24.13"
equation "\"spacerThickness\" = 2.54"
equation "\"knotHoleDepth\" = 11.1125"
body "Solid3"
